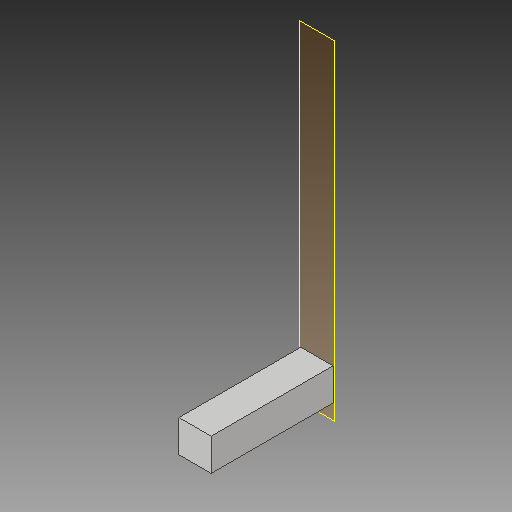
# Autodesk Inventor part: Side Frame
Saved by Autodesk Inventor 2018.1 (Build 221171000, 171)
## iProperties
Created: 2024-06-06
Part Number: Side Frame
Material: Generic
Document SubType Name: Modeling
Designer: Enrico
Density: 1 g/cm^3
Appearance: Default
Author: Enrico
Autodesk Inventor part; units mm, degrees
ref_plane "YZ Plane" through (0, 0, 0) normal (1, 0, 0) x (0, 1, 0)
ref_plane "XZ Plane" through (0, 0, 0) normal (0, 1, 0) x (-1, 0, 0)
ref_plane "Work Plane1" through (173.1259, 333.3614, 0) normal (0, 0, 1) x (0, -1, 0)
sketch "Sketch1" plane through (173.1259, 333.3614, 0) normal (0, 0, 1) x (0, -1, 0)
  line L0 (-185.9, 20) -> (185.9, 20) projected
  line L1 (185.9, 20) -> (185.9, -20) projected
  line L2 (185.9, -20) -> (-185.9, -20) projected
  line L3 (-185.9, -20) -> (-185.9, 20) projected
  line L4 (185.9, -20) -> (145.9, -20)
  line L5 (145.9, -20) -> (145.9, 20)
  line L6 (145.9, 20) -> (185.9, 20)
  line L7 (185.9, 20) -> (185.9, -20)
  point P0 (333.3614, -173.1259)
  dimension "d0" = 40
  constraints: 8 end point, 2 parallel, 1 horizontal, 1 perpendicular, 1 point on line
  measures "d0" distance between parallel lines of L1 L5
ref_plane "Work Plane2" through (-483.3514, -22, 151.3) normal (0, 0, -1) x (0, 1, 0)
extrude "Extrusion1" add sketch "Sketch1" along normal up to surface (151.3 mm away) contours L0 L1 L2 L5
body "Solid1"
